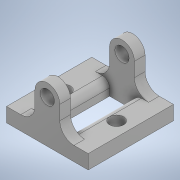
# Autodesk Inventor part: Soporte_Bomba
Saved by Autodesk Inventor 2020 (Build 240168000, 168)
## iProperties
Created: 2020-10-29
Part Number: Soporte_Bomba
Material: PC/ABS Plastic
Document SubType Name: Modeling
Designer: aaron
Density: 0.357273 g/cm^3
Appearance: Smooth - Medium Gray
Author: aaron
## iProperties of the stored document _3DPrint.ipt
Created: 2020-11-03
Part Number: _3DPrint
Material: Generic
Document SubType Name: Modeling
Designer: aaron
Density: 1 g/cm^3
Appearance: Default
Author: aaron
Autodesk Inventor part; units mm, degrees
ref_plane "YZ Plane" through (0, 0, 0) normal (1, 0, 0) x (0, 1, 0)
ref_plane "XZ Plane" through (0, 0, 0) normal (0, 1, 0) x (-1, 0, 0)
sketch "Sketch1" plane through (0, 0, 0) normal (0, 0, 1) x (1, 0, 0)
  circle A0 centre (0, 0) radius 1
  circle A1 centre (0, 0) radius 1.75
  line L0 (-1.75, 0) -> (-1.75, -4)
  line L1 (-1.75, -4) -> (-5.75, -4)
  line L2 (-5.75, -4) -> (-5.75, -6)
  line L3 (-5.75, -6) -> (0, -6)
  line L4 (0, 0) -> (0, -6)
  line L5 (1.75, 0) -> (1.75, -4)
  line L6 (1.75, -4) -> (5.75, -4)
  line L7 (5.75, -4) -> (5.75, -6)
  line L8 (5.75, -6) -> (0, -6)
  dimension "d9" = 3.5
  dimension "d8" = 2
  dimension "d10" = 4
  dimension "d11" = 4
  dimension "d12" = 2
  dimension "d13" = 5.75
  constraints: 18 end point, 4 symmetric about line, 3 perpendicular, 2 coincident, 2 vertical, 1 centre point, 3 other
  measures "d8" diameter of A0
  measures "d10" distance of L0.start L0.end
  measures "d11" distance of L0.end L1.end
  measures "d12" distance of L1.end L2.end
  measures "d13" distance of L2.end L3.end
extrude "Extrusion1" add sketch "Sketch1" along normal blind 12
ref_plane "Work Plane1" through (-5.75, 2, 0) normal (0, 1, 0) x (1, 0, 0)
sketch "Sketch2" plane through (-5.75, 2, 0) normal (0, 1, 0) x (1, 0, 0)
  line L0 (7.5, 0) -> (7.5, -12) projected
  line L1 (4, 0) -> (7.5, 0) projected
  line L2 (4, 0) -> (4, -12) projected
  line L3 (4, -12) -> (7.5, -12) projected
  line L4 (6.75, -12) -> (4.75, -12) construction
  line L5 (5.75, -12) -> (5.75, 0) construction
  line L6 (7.5, -6) -> (4, -6) construction
  line L7 (4, 0) -> (4, -12) construction
  line L8 (7.5, -10.5) -> (4, -10.5)
  line L9 (4, -10.5) -> (4, -1.5)
  line L10 (4, -1.5) -> (7.5, -1.5)
  line L11 (7.5, -1.5) -> (7.5, -10.5)
  line L12 (7.5, -10.5) -> (4, -1.5) construction
  line L13 (4, -10.5) -> (7.5, -1.5) construction
  point P0 (5.75, -6)
  dimension "d17" = 9
  constraints: 16 end point, 6 midpoint, 2 parallel, 2 perpendicular, 1 horizontal, 1 point on line
  measures "d17" distance between parallel lines of L10 L8
extrude "Extrusion2" cut sketch "Sketch2" against normal blind 12 contours L0 L8 L2 L10
fillet "Fillet1" radius 2 4 edges at (1.75, -4, 0.75) (1.75, -4, 11.25) (-1.75, -4, 0.75) (-1.75, -4, 11.25)
fillet "Fillet2" radius 1 2 edges at (1.75, -4, 6) (-1.75, -4, 6)
sketch "Sketch3" plane through (-5.75, -4, 12) normal (0, 1, 0) x (1, 0, 0)
  line L0 (8.5, 1.5) -> (8.5, 10.5) projected
  line L1 (8.5, 1.5) -> (9.5, 1.5) projected
  line L2 (9.5, 0) -> (9.5, 1.5) projected
  line L3 (11.5, 0) -> (9.5, 0) projected
  line L4 (11.5, 12) -> (11.5, 0) projected
  line L5 (11.5, 12) -> (9.5, 12) projected
  line L6 (9.5, 10.5) -> (9.5, 12) projected
  line L7 (9.5, 10.5) -> (8.5, 10.5) projected
  line L8 (3, 10.5) -> (3, 1.5) projected
  line L9 (3, 10.5) -> (2, 10.5) projected
  line L10 (2, 12) -> (2, 10.5) projected
  line L11 (2, 12) -> (0, 12) projected
  line L12 (0, 12) -> (0, 0) projected
  line L13 (2, 0) -> (0, 0) projected
  line L14 (2, 1.5) -> (2, 0) projected
  line L15 (2, 1.5) -> (3, 1.5) projected
  line L16 (11.5, 12) -> (11.5, 0) construction
  line L17 (11.5, 6) -> (0, 6) construction
  line L18 (0, 12) -> (0, 0) construction
  circle A0 centre (9.5, 6) radius 1
  circle A1 centre (2, 6) radius 1
  point P0 (5.75, 12)
  dimension "d22" = 2
  dimension "d23" = 2
  dimension "d24" = 2
  constraints: 2 centre point, 2 end point, 2 midpoint, 2 point on line, 1 equal radius
  measures "d22" diameter of A0
  measures "d23" distance from line of L4 A0.centre
  measures "d24" distance from line of L18 A1.centre
extrude "Extrusion3" cut sketch "Sketch3" against normal through all contours A0 | A1
body "Solid1"
